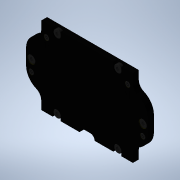
# Autodesk Inventor part: SCHUNK-5524250 Deckel-PGN-plus-P 160
Saved by Autodesk Inventor 2021 (Build 250183000, 183)
## iProperties
Created: 2025-07-30
Part Number: SCHUNK-5524250 Deckel-PGN-plus-P 160
Material: Generic
Catalog Web Link: www.cadenas.de
Description: Deckel PGN-plus-P-2-finger parallel gripper
Vendor: SCHUNK
Document SubType Name: Modeling
Designer: psAdmin
Manufacturer: SCHUNK
Mass: 38.1677 g
Surface Area: 169.217 cm^2
Volume: 38.1677 cm^3
Density: 1 g/cm^3
Appearance: PSOLRGB-128-128-64
Category: PARTsolutions
Company: SCHUNK
Title: SCHUNK-5524250 Deckel-PGN-plus-P 160
Author: Cadenas PARTsolutions
Comments: 2-finger parallel gripper
PSOL_IDENT_0: {$CADENAS_DATA/23d-libs/schunk/greifsysteme/greifmodule/greifmodule_pneumatisch/2_finger_parallelgre
PSOL_IDENT_1: ifer/2_finger_universalgreifer/pgn_plus_p/pgnplus_p_dec.prj},223 {VTYP=3D},{NB=SCHUNK-5524250 Deckel
PSOL_IDENT_2: -PGN-plus-P 160},{LINA=SCHUNK-5524250 Deckel-PGN-plus-P 160},{NN=Deckel PGN-plus-P},{DATE=24.02.2025
PSOL_IDENT_3: 16:11:11},{GEOMDATE=26.07.2024 09:17:38},{VERSION=},{LINEID=80},{WBVAR=},{WBNUMERIC=}  {NB=SCHUNK-5
PSOL_IDENT_4: 524250 Deckel-PGN-plus-P 160},{LINA=SCHUNK-5524250 Deckel-PGN-plus-P 160},{KT=DUMMY},{IDNR=5524250},
PSOL_IDENT_5: {TYP=PGN-plus-P 160},{TYP1=8.000},{L1=112.700},{B1=71.600},{H1=5.450},{L2=84.700},{R1=7.650},{R2=15.
PSOL_IDENT_6: 000},{LG1=24.500},{LG2=75.000},{G1=5.000},{G1T=4.0},{TKT=3.000},{D1=1.000},{D2=0.500},{TT=1.800},{LS
PSOL_IDENT_7: 1=64.000},{LS2=56.000},{LS3=56.000},{LS4=103.000},{LS5=0.000},{SD1=7.500},{ST1=3.200},{BA=14.000},{R
PSOL_IDENT_8: A=4.000},{TA=4.100},{DSK=7.000},{HSK=2.800},{SWS=3.000},{TSWS=1.600},{L1G=15.800},{HG=6.000},{LA=35.
PSOL_IDENT_9: 100},{LB=39.700},{L1R1=50.000},{L2R1=28.000},{L1R2=41.350},{L2R2=7.067},{DA=0.000},{WA=0.000},{A1=0.
PSOL_IDENT_10: 000},{LG3=103.000},{LG4=10.000}
NB: SCHUNK-5524250 Deckel-PGN-plus-P 160
NN: Deckel PGN-plus-P
NT: 2-finger parallel gripper
NBSYN: SCHUNK-$IDNR. Deckel-$TYP.
LINA: SCHUNK-5524250 Deckel-PGN-plus-P 160
CATALOG: SCHUNK
IDNR: 5524250
TYP: PGN-plus-P 160
TYP1: 8
L1: 112.7
B1: 71.6
H1: 5.45
L2: 84.7
R1: 7.65
R2: 15
LG1: 24.5
LG2: 75
G1: 5
G1T: 4
TKT: 3
D1: 1
D2: 0.5
TT: 1.8
LS1: 64
LS2: 56
LS3: 56
LS4: 103
LS5: 0
SD1: 7.5
ST1: 3.2
BA: 14
RA: 4
TA: 4.1
DSK: 7
HSK: 2.8
SWS: 3
TSWS: 1.6
L1G: 15.8
HG: 6
LA: 35.1
LB: 39.7
L1R1: 50
L2R1: 28
L1R2: 41.35
L2R2: 7.067
DA: 0
WA: 0
A1: 0
LG3: 103
LG4: 10
SUPPLIER: SCHUNK
ARTICLENO: SCHUNK-5524250 Deckel-PGN-plus-P 160
BOMINFO: SCHUNK-5524250 Deckel-PGN-plus-P 160
CREATOR: CADENAS GmbH
Autodesk Inventor part; units mm, degrees
sketch "Sketch_36" plane through (0, 0, 0) normal (0, 0, 1) x (1, 0, 0)
  line L0 (-56.35, 7.067) -> (-56.35, -7.067)
  arc A0 (-56.35, -7.067) -> (-47.0785, -20.9301) centre (-41.35, -7.067) ccw
  arc A1 (-42.35, -28.0002) -> (-47.0785, -20.9301) centre (-50, -28.0002) ccw
  line L1 (-42.35, -28.0002) -> (-42.35, -35.8)
  line L2 (-42.35, -35.8) -> (42.35, -35.8)
  line L3 (42.35, -35.8) -> (42.35, -28.0002)
  arc A2 (47.0785, -20.9301) -> (42.35, -28.0002) centre (50, -28.0002) ccw
  arc A3 (47.0785, -20.9301) -> (56.35, -7.067) centre (41.35, -7.067) ccw
  line L4 (56.35, -7.067) -> (56.35, 7.067)
  arc A4 (56.35, 7.067) -> (47.0785, 20.9301) centre (41.35, 7.067) ccw
  arc A5 (42.35, 28.0002) -> (47.0785, 20.9301) centre (50, 28.0002) ccw
  line L5 (42.35, 28.0002) -> (42.35, 35.8)
  line L6 (42.35, 35.8) -> (-42.35, 35.8)
  line L7 (-42.35, 35.8) -> (-42.35, 28.0002)
  arc A6 (-47.0785, 20.9301) -> (-42.35, 28.0002) centre (-50, 28.0002) ccw
  arc A7 (-47.0785, 20.9301) -> (-56.35, 7.067) centre (-41.35, 7.067) ccw
  constraints: 16 end point, 16 point on circle, 8 centre point
extrude "Extrusion1" add sketch "Sketch_36" along normal blind 5.45
sketch "Sketch_3" plane through (0, 24.5, 0) normal (0, 1, 0) x (1, 0, 0)
  line L0 (37.5, -5.45) -> (37.5, -5.35)
  line L1 (37.5, -5.35) -> (39.7279, -5.35)
  line L2 (39.7279, -5.35) -> (40, -5.0779)
  line L3 (40, -5.0779) -> (40, -5.45)
  line L4 (40, -5.45) -> (37.5, -5.45)
  line L5 (37.5, -5.45) -> (37.5, -5.35)
  constraints: 12 end point
revolve "Revolution1" cut sketch "Sketch_3" angle 360 about axis through (37.5, 24.5, 5.45) along (0, 0, 1)
pattern_linear "Rectangular Pattern1" count 2 spacing 75 along (-1, 0, 0) of "Revolution1"
sketch "Sketch_5" plane through (0, 0, 5.45) normal (0, 0, 1) x (1, 0, 0)
  arc A0 (36.25, 24.067) -> (36.5, 23.634) centre (36.375, 23.8505) ccw
  arc A1 (37.25, 23.201) -> (36.5, 23.634) centre (36.75, 23.201) ccw
  arc A2 (37.25, 23.201) -> (37.75, 23.201) centre (37.5, 23.201) ccw
  arc A3 (38.5, 23.634) -> (37.75, 23.201) centre (38.25, 23.201) ccw
  arc A4 (38.5, 23.634) -> (38.75, 24.067) centre (38.625, 23.8505) ccw
  arc A5 (38.75, 24.933) -> (38.75, 24.067) centre (39, 24.5) ccw
  arc A6 (38.75, 24.933) -> (38.5, 25.366) centre (38.625, 25.1495) ccw
  arc A7 (37.75, 25.799) -> (38.5, 25.366) centre (38.25, 25.799) ccw
  arc A8 (37.75, 25.799) -> (37.25, 25.799) centre (37.5, 25.799) ccw
  arc A9 (36.5, 25.366) -> (37.25, 25.799) centre (36.75, 25.799) ccw
  arc A10 (36.5, 25.366) -> (36.25, 24.933) centre (36.375, 25.1495) ccw
  arc A11 (36.25, 24.067) -> (36.25, 24.933) centre (36, 24.5) ccw
  constraints: 24 point on circle, 12 centre point
extrude "Extrusion2" cut sketch "Sketch_5" against normal blind 1.8
pattern_linear "Rectangular Pattern2" count 2 spacing 75 along (-1, 0, 0) of "Extrusion2"
sketch "Sketch_43" plane through (0, -10, 0) normal (0, 1, 0) x (1, 0, 0)
  line L0 (51.5, -5.45) -> (51.5, -5.35)
  line L1 (51.5, -5.35) -> (53.7279, -5.35)
  line L2 (53.7279, -5.35) -> (54, -5.0779)
  line L3 (54, -5.0779) -> (54, -5.45)
  line L4 (54, -5.45) -> (51.5, -5.45)
  line L5 (51.5, -5.45) -> (51.5, -5.35)
  constraints: 12 end point
revolve "Revolution2" cut sketch "Sketch_43" angle 360 about axis through (51.5, -10, 5.45) along (0, 0, 1)
pattern_linear "Rectangular Pattern3" count 2 spacing 103 along (-1, 0, 0) of "Revolution2"
sketch "Sketch_45" plane through (0, 0, 5.45) normal (0, 0, 1) x (1, 0, 0)
  arc A0 (50.25, -10.433) -> (50.5, -10.866) centre (50.375, -10.6495) ccw
  arc A1 (51.25, -11.299) -> (50.5, -10.866) centre (50.75, -11.299) ccw
  arc A2 (51.25, -11.299) -> (51.75, -11.299) centre (51.5, -11.299) ccw
  arc A3 (52.5, -10.866) -> (51.75, -11.299) centre (52.25, -11.299) ccw
  arc A4 (52.5, -10.866) -> (52.75, -10.433) centre (52.625, -10.6495) ccw
  arc A5 (52.75, -9.567) -> (52.75, -10.433) centre (53, -10) ccw
  arc A6 (52.75, -9.567) -> (52.5, -9.134) centre (52.625, -9.3505) ccw
  arc A7 (51.75, -8.701) -> (52.5, -9.134) centre (52.25, -8.701) ccw
  arc A8 (51.75, -8.701) -> (51.25, -8.701) centre (51.5, -8.701) ccw
  arc A9 (50.5, -9.134) -> (51.25, -8.701) centre (50.75, -8.701) ccw
  arc A10 (50.5, -9.134) -> (50.25, -9.567) centre (50.375, -9.3505) ccw
  arc A11 (50.25, -10.433) -> (50.25, -9.567) centre (50, -10) ccw
  constraints: 24 point on circle, 12 centre point
extrude "Extrusion3" cut sketch "Sketch_45" against normal blind 3.2
pattern_linear "Rectangular Pattern4" count 2 spacing 103 along (-1, 0, 0) of "Extrusion3"
sketch "Sketch_53" plane through (0, 0, 5.45) normal (0, 0, 1) x (1, 0, 0)
  line L0 (24.25, -32) -> (24.25, -35.8)
  line L1 (24.25, -35.8) -> (31.75, -35.8)
  line L2 (31.75, -35.8) -> (31.75, -32)
  arc A0 (31.75, -32) -> (24.25, -32) centre (28, -32) ccw
  constraints: 6 end point, 2 point on circle, 1 centre point
extrude "Extrusion4" cut sketch "Sketch_53" against normal blind 3.2
pattern_linear "Rectangular Pattern5" count 2 spacing 56 along (-1, 0, 0) of "Extrusion4"
sketch "Sketch_55" plane through (0, 0, 5.45) normal (0, 0, 1) x (1, 0, 0)
  arc A0 (24.25, 32) -> (31.75, 32) centre (28, 32) ccw
  line L0 (31.75, 32) -> (31.75, 35.8)
  line L1 (31.75, 35.8) -> (24.25, 35.8)
  line L2 (24.25, 35.8) -> (24.25, 32)
  constraints: 6 end point, 2 point on circle, 1 centre point
extrude "Extrusion5" cut sketch "Sketch_55" against normal blind 3.2
pattern_linear "Rectangular Pattern6" count 2 spacing 56 along (-1, 0, 0) of "Extrusion5"
sketch "Sketch8" plane through (0, 0, 5.45) normal (0, 0, 1) x (1, 0, 0)
  point P0 (51.5, 0)
hole "Hole1" at (51.5, 0, 5.45) direction (0, 0, -1) diameter 7.5 depth 3.2
pattern_linear "Rectangular Pattern7" count 2 spacing 103 along (-1, 0, 0) of "Hole1"
sketch "Sketch_52" plane through (0, 0, 0) normal (0, 0, 1) x (1, 0, 0)
  line L0 (-7, -35.7) -> (-7, -35.8)
  line L1 (-7, -35.8) -> (7, -35.8)
  line L2 (7, -35.8) -> (7, -35.7)
  arc A0 (7, -35.7) -> (3, -31.7) centre (3, -35.7) ccw
  line L3 (3, -31.7) -> (-3, -31.7)
  arc A1 (-3, -31.7) -> (-7, -35.7) centre (-3, -35.7) ccw
  constraints: 8 end point, 4 point on circle, 2 centre point
extrude "Extrusion6" cut sketch "Sketch_52" along normal blind 5.45
sketch "Sketch_13" plane through (0, 32, 0) normal (0, 1, 0) x (1, 0, 0)
  line L0 (28, -5.05) -> (28, -2.25)
  line L1 (28, -2.25) -> (31.5, -2.25)
  line L2 (31.5, -2.25) -> (31.5, -4.75)
  arc A0 (31.2, -5.05) -> (31.5, -4.75) centre (31.2, -4.75) ccw
  line L3 (31.2, -5.05) -> (28, -5.05)
  line L4 (28, -5.05) -> (28, -2.25)
  constraints: 10 end point, 2 point on circle, 1 centre point
revolve "Revolution3" add sketch "Sketch_13" angle 360 about axis through (28, 32, 5.05) along (0, 0, 1)
pattern_linear "Rectangular Pattern8" count 2 spacing 56 along (-1, 0, 0) count 2 spacing 64 along (0, -1, 0) of "Revolution3"
sketch "Sketch_15" plane through (0, 0, 5.05) normal (0, 0, 1) x (1, 0, 0)
  line L0 (26.5, 31.134) -> (28, 30.2679)
  line L1 (28, 30.2679) -> (29.5, 31.134)
  line L2 (29.5, 31.134) -> (29.5, 32.866)
  line L3 (29.5, 32.866) -> (28, 33.7321)
  line L4 (28, 33.7321) -> (26.5, 32.866)
  line L5 (26.5, 32.866) -> (26.5, 31.134)
  constraints: 12 end point
extrude "Extrusion7" cut sketch "Sketch_15" against normal blind 1.6
pattern_linear "Rectangular Pattern9" count 2 spacing 56 along (-1, 0, 0) count 2 spacing 64 along (0, -1, 0) of "Extrusion7"
sketch "Sketch_26" plane through (0, 0, 0) normal (0, 1, 0) x (-1, 0, 0)
  line L0 (-51.5, 5.05) -> (-51.5, 2.25)
  line L1 (-51.5, 2.25) -> (-55, 2.25)
  line L2 (-55, 2.25) -> (-55, 4.75)
  arc A0 (-54.7, 5.05) -> (-55, 4.75) centre (-54.7, 4.75) ccw
  line L3 (-54.7, 5.05) -> (-51.5, 5.05)
  line L4 (-51.5, 5.05) -> (-51.5, 2.25)
  constraints: 10 end point, 2 point on circle, 1 centre point
revolve "Revolution4" add sketch "Sketch_26" angle 360 about axis through (51.5, 0, 5.05) along (0, 0, 1)
pattern_linear "Rectangular Pattern10" count 2 spacing 103 along (-1, 0, 0) of "Revolution4"
sketch "Sketch_28" plane through (0, 0, 5.05) normal (0, 0, 1) x (1, 0, 0)
  line L0 (50, -0.866) -> (51.5, -1.7321)
  line L1 (51.5, -1.7321) -> (53, -0.866)
  line L2 (53, -0.866) -> (53, 0.866)
  line L3 (53, 0.866) -> (51.5, 1.7321)
  line L4 (51.5, 1.7321) -> (50, 0.866)
  line L5 (50, 0.866) -> (50, -0.866)
  constraints: 12 end point
extrude "Extrusion8" cut sketch "Sketch_28" against normal blind 1.6
pattern_linear "Rectangular Pattern11" count 2 spacing 103 along (-1, 0, 0) of "Extrusion8"
sketch "Sketch_47" plane through (0, 0, 5.45) normal (0, 0, 1) x (1, 0, 0)
  line L0 (-39.1, 20) -> (-38.974, 19.616)
  line L1 (-38.974, 19.616) -> (-38.85, 18.978)
  line L2 (-38.85, 18.978) -> (-38.85, 16.936)
  line L3 (-38.85, 16.936) -> (-38.724, 16.552)
  line L4 (-38.724, 16.552) -> (-38.474, 16.298)
  line L5 (-38.474, 16.298) -> (-38.1, 16.042)
  line L6 (-38.1, 16.042) -> (-37.35, 15.914)
  line L7 (-37.35, 15.914) -> (-36.6, 15.914)
  line L8 (-36.6, 15.914) -> (-35.724, 16.042)
  line L9 (-35.724, 16.042) -> (-35.474, 16.17)
  line L10 (-35.474, 16.17) -> (-35.224, 16.426)
  line L11 (-35.224, 16.426) -> (-35.1, 16.68)
  line L12 (-35.1, 16.68) -> (-35.1, 16.936)
  line L13 (-35.1, 16.936) -> (-35.724, 16.936)
  line L14 (-35.724, 16.936) -> (-35.85, 16.68)
  line L15 (-35.85, 16.68) -> (-36.1, 16.552)
  line L16 (-36.1, 16.552) -> (-36.6, 16.426)
  line L17 (-36.6, 16.426) -> (-37.35, 16.426)
  line L18 (-37.35, 16.426) -> (-37.85, 16.552)
  line L19 (-37.85, 16.552) -> (-38.1, 16.68)
  line L20 (-38.1, 16.68) -> (-38.224, 16.936)
  line L21 (-38.224, 16.936) -> (-38.224, 17.318)
  line L22 (-38.224, 17.318) -> (-36.85, 17.318)
  line L23 (-36.85, 17.318) -> (-36.1, 17.446)
  line L24 (-36.1, 17.446) -> (-35.6, 17.702)
  line L25 (-35.6, 17.702) -> (-35.35, 17.956)
  line L26 (-35.35, 17.956) -> (-35.1, 18.468)
  line L27 (-35.1, 18.468) -> (-35.1, 18.85)
  line L28 (-35.1, 18.85) -> (-35.224, 19.362)
  line L29 (-35.224, 19.362) -> (-35.6, 19.744)
  line L30 (-35.6, 19.744) -> (-35.85, 19.872)
  line L31 (-35.85, 19.872) -> (-36.35, 20)
  line L32 (-36.35, 20) -> (-37.1, 20)
  line L33 (-37.1, 20) -> (-37.724, 19.872)
  line L34 (-37.724, 19.872) -> (-38.1, 19.616)
  line L35 (-38.1, 19.616) -> (-38.224, 19.362)
  line L36 (-38.224, 19.362) -> (-38.35, 19.744)
  line L37 (-38.35, 19.744) -> (-38.474, 20)
  line L38 (-38.474, 20) -> (-39.1, 20)
  line L39 (-38.224, 17.83) -> (-36.85, 17.83)
  line L40 (-36.85, 17.83) -> (-36.35, 17.956)
  line L41 (-36.35, 17.956) -> (-36.1, 18.084)
  line L42 (-36.1, 18.084) -> (-35.85, 18.34)
  line L43 (-35.85, 18.34) -> (-35.724, 18.722)
  line L44 (-35.724, 18.722) -> (-35.724, 18.978)
  line L45 (-35.724, 18.978) -> (-35.85, 19.234)
  line L46 (-35.85, 19.234) -> (-36.35, 19.488)
  line L47 (-36.35, 19.488) -> (-37.1, 19.488)
  line L48 (-37.1, 19.488) -> (-37.724, 19.234)
  line L49 (-37.724, 19.234) -> (-38.1, 18.85)
  line L50 (-38.1, 18.85) -> (-38.224, 18.596)
  line L51 (-38.224, 18.596) -> (-38.224, 17.83)
  constraints: 104 end point
extrude "Extrusion9" cut sketch "Sketch_47" against normal blind 0.3
sketch "Sketch_48" plane through (0, 0, 5.45) normal (0, 0, 1) x (1, 0, 0)
  line L0 (35.7, 18.468) -> (35.7, 17.446)
  line L1 (35.7, 17.446) -> (35.826, 16.936)
  line L2 (35.826, 16.936) -> (35.95, 16.68)
  line L3 (35.95, 16.68) -> (36.326, 16.298)
  line L4 (36.326, 16.298) -> (36.7, 16.042)
  line L5 (36.7, 16.042) -> (37.2, 15.914)
  line L6 (37.2, 15.914) -> (37.95, 15.914)
  line L7 (37.95, 15.914) -> (38.45, 16.042)
  line L8 (38.45, 16.042) -> (38.7, 16.17)
  line L9 (38.7, 16.17) -> (38.95, 16.426)
  line L10 (38.95, 16.426) -> (39.076, 16.68)
  line L11 (39.076, 16.68) -> (39.076, 14)
  line L12 (39.076, 14) -> (39.7, 14)
  line L13 (39.7, 14) -> (39.7, 20)
  line L14 (39.7, 20) -> (39.076, 20)
  line L15 (39.076, 20) -> (39.076, 19.234)
  line L16 (39.076, 19.234) -> (38.95, 19.488)
  line L17 (38.95, 19.488) -> (38.7, 19.744)
  line L18 (38.7, 19.744) -> (38.45, 19.872)
  line L19 (38.45, 19.872) -> (37.95, 20)
  line L20 (37.95, 20) -> (37.2, 20)
  line L21 (37.2, 20) -> (36.7, 19.872)
  line L22 (36.7, 19.872) -> (36.326, 19.616)
  line L23 (36.326, 19.616) -> (35.826, 18.978)
  line L24 (35.826, 18.978) -> (35.7, 18.468)
  line L25 (36.326, 18.34) -> (36.326, 17.574)
  line L26 (36.326, 17.574) -> (36.45, 17.19)
  line L27 (36.45, 17.19) -> (36.7, 16.808)
  line L28 (36.7, 16.808) -> (37.2, 16.552)
  line L29 (37.2, 16.552) -> (37.95, 16.552)
  line L30 (37.95, 16.552) -> (38.45, 16.68)
  line L31 (38.45, 16.68) -> (38.826, 16.936)
  line L32 (38.826, 16.936) -> (39.076, 17.318)
  line L33 (39.076, 17.318) -> (39.076, 18.596)
  line L34 (39.076, 18.596) -> (38.826, 18.978)
  line L35 (38.826, 18.978) -> (38.45, 19.234)
  line L36 (38.45, 19.234) -> (37.95, 19.362)
  line L37 (37.95, 19.362) -> (37.45, 19.362)
  line L38 (37.45, 19.362) -> (36.95, 19.234)
  line L39 (36.95, 19.234) -> (36.576, 18.978)
  line L40 (36.576, 18.978) -> (36.326, 18.34)
  constraints: 82 end point
extrude "Extrusion10" cut sketch "Sketch_48" against normal blind 0.2
ref_plane "einbau_XY" through (0, 0, 0) normal (0, 0, 1) x (1, 0, 0)
ref_plane "einbau_YZ" through (0, 0, 0) normal (1, 0, 0) x (0, 1, 0)
ref_plane "einbau_ZX" through (0, 0, 0) normal (0, 1, 0) x (0, 0, 1)
body "Solid1"
